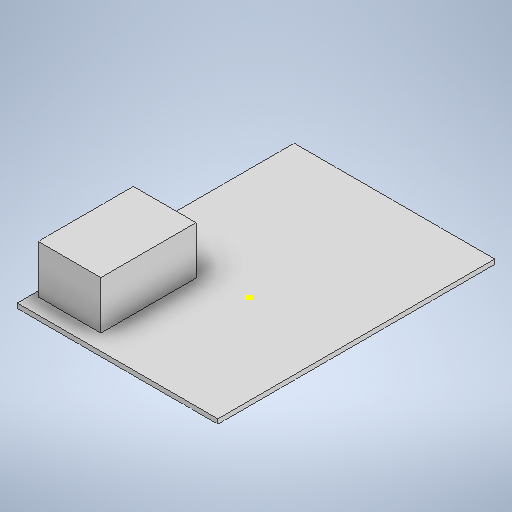
# Autodesk Inventor part: Board
Saved by Autodesk Inventor 2025 (Build 290162000, 162)
## iProperties
Created: 2024-10-01
Part Number: Board
Material: Generic
Document SubType Name: Modeling
Designer: willi
Density: 1 g/cm^3
Appearance: Default
Author: willi
Autodesk Inventor part; units mm, degrees
ref_plane "YZ Plane" through (0, 0, 0) normal (1, 0, 0) x (0, 1, 0)
ref_plane "XZ Plane" through (0, 0, 0) normal (0, 1, 0) x (-1, 0, 0)
ref_plane "XY Plane" through (0, 0, 0) normal (0, 0, 1) x (1, 0, 0)
sketch "Sketch1" plane through (0, 0, 0) normal (0, 1, 0) x (-1, 0, 0)
  line L0 (39.8244, 42.085) -> (-31.1756, 42.085)
  line L1 (-31.1756, 42.085) -> (-31.1756, -55.915)
  line L2 (-31.1756, -55.915) -> (39.8244, -55.915)
  line L3 (39.8244, -55.915) -> (39.8244, 42.085)
  point P0 (0, 0)
  dimension "d0" = 71
  dimension "d1" = 98
  constraints: 8 end point, 2 parallel, 1 horizontal, 1 perpendicular
  measures "d0" distance between parallel lines of L1 L3
  measures "d1" distance between parallel lines of L2 L0
extrude "Extrusion1" add sketch "Sketch1" along normal blind 1.66
sketch "Sketch2" plane through (0, 1.66, 0) normal (0, 1, 0) x (1, 0, 0)
  line L0 (-38.0351, -2.7975) -> (-15.8351, -2.7975)
  line L1 (-15.8351, -2.7975) -> (-15.8351, -36.4975)
  line L2 (-15.8351, -36.4975) -> (-38.0351, -36.4975)
  line L3 (-38.0351, -36.4975) -> (-38.0351, -2.7975)
  point P0 (0, 0)
  dimension "d4" = 33.7
  dimension "d5" = 22.2
  constraints: 8 end point, 2 parallel, 1 horizontal, 1 perpendicular
  measures "d4" distance of L0.end L1.end
  measures "d5" distance of L0.start L0.end
extrude "Extrusion2" add sketch "Sketch2" along normal blind 17
sketch "Sketch3" plane through (0, 1.66, 0) normal (0, 1, 0) x (1, 0, 0)
  point P0 (0, 0)
body "Solid1"
